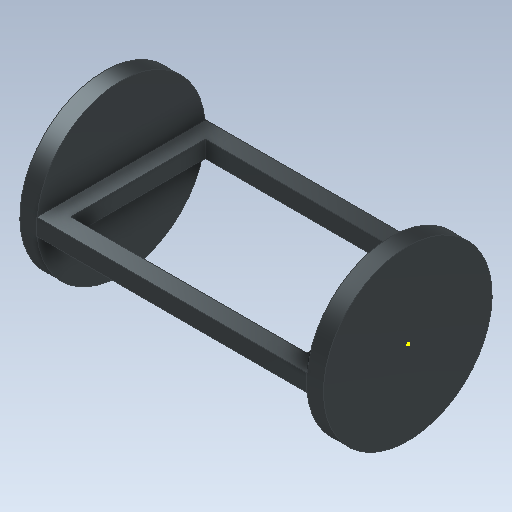
# Autodesk Inventor part: electronicsbay
Saved by Autodesk Inventor 2020.3 (Build 243373000, 373)
## iProperties
Created: 2021-03-10
Part Number: electronicsbay
Material: ABS Plastic
Document SubType Name: Modeling
Designer: 0x6f736f646f
Density: 1.06 g/cm^3
Appearance: Iron Gray
Mass: 27.2195 g
Surface Area: 132.427 cm^2
Volume: 25.6788 cm^3
Author: 0x6f736f646f
Autodesk Inventor part; units mm, degrees
ref_plane "YZ Plane" through (0, 0, 0) normal (1, 0, 0) x (0, 1, 0)
ref_plane "XZ Plane" through (0, 0, 0) normal (0, 1, 0) x (-1, 0, 0)
ref_plane "XY Plane" through (0, 0, 0) normal (0, 0, 1) x (1, 0, 0)
sketch "Sketch1" plane through (0, 0, 0) normal (0, 1, 0) x (-1, 0, 0)
  point P0 (0, 0)
sketch "Sketch2" plane through (0, 0, 0) normal (0, 0, 1) x (1, 0, 0)
  line L0 (0, 0) -> (0, 25)
  line L1 (0, 25) -> (-5, 25)
  line L2 (-5, 25) -> (-5, 2.5)
  line L3 (-5, 2.5) -> (-85, 2.5)
  line L4 (-85, 2.5) -> (-85, 25)
  line L5 (-85, 25) -> (-90, 25)
  line L6 (-90, 25) -> (-90, 0)
  line L7 (-90, 0) -> (0, 0)
  line L8 (-85, 2.5) -> (-5, 2.5)
  line L9 (-5, 2.5) -> (-5, -2.5)
  line L10 (-5, -2.5) -> (-85, -2.5)
  line L11 (-85, -2.5) -> (-85, 2.5)
  dimension "d0" = 25
  dimension "d1" = 5
  dimension "d2" = 22.5
  dimension "d3" = 80
  dimension "d4" = 5
  dimension "d6" = 5
  constraints: 24 end point, 7 perpendicular, 2 parallel, 2 point on line, 1 horizontal, 1 vertical
  measures "d0" distance of L0.start L0.end
  measures "d1" distance of L0.end L1.end
  measures "d2" distance of L1.end L2.end
  measures "d3" distance of L2.end L3.end
  measures "d4" distance of L4.end L5.end
  measures "d6" distance of L8.end L9.end
revolve "Revolution1" add sketch "Sketch2" angle 360 about axis through (-90, 0, 0) along (1, 0, 0) contours L7 L9 L2 L1 L0 | L7 L11 L3 L9 | L7 L6 L5 L4 L11
extrude "Extrusion1" add sketch "Sketch2" along normal mid plane 50 contours L9 L10 L11 L7 | L7 L11 L3 L9
sketch "Sketch3" plane through (-85, 2.5, -25) normal (0, 1, 0) x (1, 0, 0)
  line L0 (80, 0) -> (0, 0) projected
  line L1 (80, -49.8747) -> (80, -0.1253) projected
  line L2 (0, 0) -> (80, 0)
  line L3 (80, 0) -> (80, -49.8747)
  line L4 (80, -49.8747) -> (0, -49.8747)
  line L5 (0, -49.8747) -> (0, 0)
  line L6 (5, -5) -> (75, -5)
  line L7 (75, -5) -> (75, -44.8747)
  line L8 (75, -44.8747) -> (5, -44.8747)
  line L9 (5, -44.8747) -> (5, -5)
  point P0 (85, -25)
  dimension "d9" = 5
  constraints: 16 end point, 4 parallel, 2 perpendicular, 1 horizontal, 3 other
  measures "d9" distance between parallel lines of L5 L9
extrude "Extrusion2" cut sketch "Sketch3" against normal mid plane 20 contours L6 L7 L8 L9
body "Solid1"
